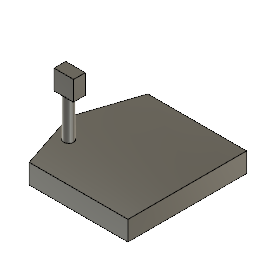
Robotic arm( ball throwing) (Autodesk Fusion 360 archive; units mm, degrees)
design "ra2 1"
Autodesk Fusion 360 part; units mm, degrees
sketch "Sketch1" plane through (0, 0, 0) normal (0, 0, 1) x (1, 0, 0)
  line L0 (0, 300) -> (500, 300)
  line L1 (0, -300) -> (500, -300)
  line L2 (0, 300) -> (-100, 0)
  line L3 (-100, 0) -> (0, -300)
  line L4 (500, 300) -> (500, -300)
  dimension "d1" = 500
  constraint horizontal L0
  constraint perpendicular L1 L4
  measures "d1" distance of L0.start L0.end
extrude "Extrude1" add sketch "Sketch1" along normal blind 100
sketch "Sketch2" plane through (0, 0, 100) normal (0, 0, 1) x (-1, 0, 0)
  line L0 (0, -300) -> (100, 0)
  line L1 (100, 0) -> (0, 300)
  line L2 (0, 300) -> (-500, 300)
  line L3 (-500, 300) -> (-500, -300)
  line L4 (-500, -300) -> (0, -300)
  circle A0 centre (0, 100) radius 25
  circle A1 centre (0, -100) radius 25
  dimension "d7" = 50
  dimension "d8" = 50
  measures "d7" diameter of A0
  measures "d8" diameter of A1
extrude "Extrude2" add sketch "Sketch2" along normal blind 265 contours A0
ref_plane "WorkPlane1" through (0, -125, 274.5445) normal (0, -1, 0) x (-1, 0, 0)
sketch "Sketch3" plane through (0, -125, 0) normal (0, -1, 0) x (-1, 0, 0)
  line L0 (50, -300) -> (-50, -300)
  line L1 (-50, -300) -> (-50, -400)
  line L2 (-50, -400) -> (50, -400)
  line L3 (50, -400) -> (50, -300)
  constraint horizontal L0
  constraint perpendicular L0 L1
  constraint perpendicular L1 L2
  constraint perpendicular L0 L3
extrude "Extrude3" add sketch "Sketch3" against normal blind 60
sketch "Sketch4" plane through (0, -65, 0) normal (0, 1, 0) x (-1, 0, 0)
  line L0 (50, 300) -> (50, 400)
  line L1 (50, 400) -> (-50, 400)
  line L2 (-50, 400) -> (-50, 300)
  line L3 (-50, 300) -> (50, 300)
  circle A0 centre (0, 350) radius 15
  dimension "d14" = 30
  measures "d14" diameter of A0
extrude "Extrude4" add sketch "Sketch4" along normal blind 10 contours A0
